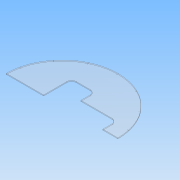
# Autodesk Inventor part: Top_Guard 2
Saved by Autodesk Inventor 2018.1 (Build 221171000, 171)
## iProperties
Created: 2019-03-23
Part Number: Top_Guard 2
Material: PMMA Plastic
Document SubType Name: Modeling
Designer: James
Density: 1.188 g/cm^3
Appearance: Polycarbonate - Clear
Author: James
Autodesk Inventor part; units mm, degrees
ref_plane "YZ Plane" through (0, 0, 0) normal (1, 0, 0) x (0, 1, 0)
ref_plane "XZ Plane" through (0, 0, 0) normal (0, 1, 0) x (-1, 0, 0)
sketch "Sketch1" plane through (0, 0, 0) normal (0, 0, 1) x (1, 0, 0)
  arc A0 (600, 0) -> (-600, 0) centre (0, 0) ccw
  line L0 (-600, 0) -> (600, 0)
  point P0 (0, 0)
  dimension "d0" = 1200
  constraints: 2 end point, 2 horizontal alignment, 2 point on circle, 1 centre point, 1 coincident, 1 horizontal, 1 midpoint
  measures "d0" distance of L0.start L0.end
extrude "Extrusion1" add sketch "Sketch1" along normal blind 10
sketch "Sketch2" plane through (0, 0, 10) normal (0, 0, 1) x (1, 0, 0)
  line L0 (-600, 0) -> (600, 0) projected
  line L1 (438, 0) -> (-198, 0)
  line L2 (-198, 0) -> (-198, 300)
  line L3 (-198, 300) -> (438, 300)
  line L4 (438, 300) -> (438, 0)
  point P0 (0, 0)
  dimension "d3" = 300
  dimension "d4" = 636
  dimension "d5" = 198
  constraints: 8 end point, 2 parallel, 1 horizontal, 1 perpendicular, 1 point on line
  measures "d3" distance of L3.end L1.start
  measures "d4" distance of L2.end L3.end
  measures "d5" distance from line of L2 point (0, 0)
extrude "Extrusion2" cut sketch "Sketch2" against normal through all
sketch "Sketch3" plane through (0, 0, 10) normal (0, 0, 1) x (1, 0, 0)
  line L0 (-198, 300) -> (438, 300) projected
  line L1 (438, 300) -> (52, 300)
  line L2 (52, 300) -> (52, 150)
  line L3 (52, 150) -> (438, 150)
  line L4 (438, 150) -> (438, 300)
  line L5 (-198, 0) -> (-198, 300) projected
  point P0 (0, 0)
  dimension "d9" = 150
  dimension "d10" = 250
  constraints: 8 end point, 2 parallel, 1 horizontal, 1 perpendicular
  measures "d9" distance of L3.end L0.end
  measures "d10" distance between parallel lines of L5 L2
extrude "Extrusion3" add sketch "Sketch3" against normal up to surface (10 mm away)
fillet "Fillet2" radius 50 3 edges at (-198, 300, 5) (52, 300, 5) (438, 150, 5)
ref_plane "Work Plane1" through (-600, 600, 0) normal (0, -1, 0) x (1, 0, 0)
sketch "Sketch4" plane through (-600, 600, 0) normal (0, -1, 0) x (1, 0, 0)
  line L0 (1200, 10) -> (0, 10) projected
  line L1 (600, 12) -> (600, -2) projected
  point P0 (600, 0)
  point P1 (600, 5)
  dimension "d15" = 5
  constraints: 1 midpoint
  measures "d15" distance from line of point (600, 5) L0
hole "Hole1" at (0, 600, 5) direction (0, -1, 0) diameter 3.242 depth 11.8 tip angle 118 thread size "M4x0.7" class "6H" standard "ANSI Metric M Profile"
pattern_circular "Circular Pattern1" count 14 over 360 about axis through (0, 0, -10) along (0, 0, 1) of "Hole1"
body "Solid1"
